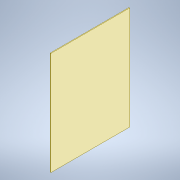
# Autodesk Inventor part: cover side
Saved by Autodesk Inventor 2021 (Build 250183000, 183)
## iProperties
Created: 2024-06-13
Part Number: cover side
Material: Nylon 6/6
Document SubType Name: Modeling
Designer: ASUS
Density: 1.13 g/cm^3
Appearance: Nylon 6
Author: ASUS
Autodesk Inventor part; units mm, degrees
ref_plane "YZ Plane" through (0, 0, 0) normal (1, 0, 0) x (0, 1, 0)
ref_plane "XZ Plane" through (0, 0, 0) normal (0, 1, 0) x (-1, 0, 0)
ref_plane "XY Plane" through (0, 0, 0) normal (0, 0, 1) x (1, 0, 0)
sketch "Sketch1" plane through (0, 0, 0) normal (1, 0, 0) x (0, 1, 0)
  line L0 (0, 0) -> (427, 0)
  line L1 (427, 0) -> (427, -326)
  line L2 (427, -326) -> (0, -326)
  line L3 (0, -326) -> (0, 0)
  dimension "d0" = 427
  dimension "d1" = 326
  constraints: 8 end point, 2 parallel, 1 horizontal, 1 perpendicular
  measures "d0" distance between parallel lines of L3 L1
  measures "d1" distance between parallel lines of L2 L0
extrude "Extrusion1" add sketch "Sketch1" along normal blind 3
body "Solid1"
